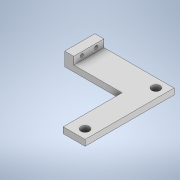
# Autodesk Inventor part: limit_switch_lower_mount
Saved by Autodesk Inventor 2022 (Build 260153000, 153)
## iProperties
Created: 2022-02-08
Part Number: limit_switch_lower_mount
Material: Generic
Document SubType Name: Modeling
Designer: kylem
Density: 1 g/cm^3
Appearance: Default
Author: kylem
Autodesk Inventor part; units mm, degrees
ref_plane "YZ Plane" through (0, 0, 0) normal (1, 0, 0) x (0, 1, 0)
ref_plane "XZ Plane" through (0, 0, 0) normal (0, 1, 0) x (-1, 0, 0)
ref_plane "XY Plane" through (0, 0, 0) normal (0, 0, 1) x (1, 0, 0)
sketch "Sketch1" plane through (0, 0, 0) normal (0, 1, 0) x (-1, 0, 0)
  line L0 (0, 0) -> (40.5, 0)
  line L1 (40.5, 0) -> (40.5, -47)
  line L2 (40.5, -47) -> (0, -47)
  line L3 (0, -47) -> (0, 0)
  circle A0 centre (0, 0) radius 2.8
  circle A1 centre (0, -47) radius 2.8
  line L4 (0, 0) -> (-6, 0)
  line L5 (-6, 0) -> (-6, 6)
  line L6 (0, -47) -> (-6, -47)
  line L7 (-6, -47) -> (-6, -53)
  line L8 (-6, -53) -> (40.5, -53)
  line L9 (40.5, -53) -> (-6, -53)
  line L10 (-6, -53) -> (-6, 6)
  line L11 (-6, 6) -> (40.5, 6)
  line L12 (40.5, 6) -> (40.5, -53)
  line L13 (40.5, 6) -> (46.5, 6)
  line L14 (46.5, 6) -> (46.5, -53)
  line L15 (46.5, -53) -> (40.5, -53)
  line L16 (40.5, -53) -> (40.5, 6)
  dimension "d0" = 40.5
  dimension "d1" = 47
  dimension "d2" = 5.6
  dimension "d3" = 5.6
  dimension "d4" = 6
  dimension "d5" = 6
  dimension "d6" = 6
  dimension "d7" = 6
  dimension "d8" = 6
  constraints: 34 end point, 7 perpendicular, 6 parallel, 4 horizontal, 2 centre point, 2 coincident, 1 point on line
  measures "d0" distance of L1.end L2.end
  measures "d1" distance of L0.end L1.end
  measures "d2" diameter of A0
  measures "d3" diameter of A1
  measures "d4" distance of L4.start L4.end
  measures "d5" distance of L4.end L5.end
  measures "d6" distance of L6.start L6.end
  measures "d7" distance of L6.end L7.end
  measures "d8" distance of L14.end L15.end
extrude "Extrusion1" add sketch "Sketch1" along normal blind 4 contours A0 L4 L5 L11 L12 L0 | L0 L1 L2 A1 L3 A0 | L3 A1 L6 L10 L4 A0 | L12 L13 L14 L15 L1 | L12 L8 L7 L6 A1 L2
sketch "Sketch3" plane through (-46.5, 0, -53) normal (-1, 0, 0) x (0, 0, 1)
  line L0 (0, 0) -> (0, 4) projected
  line L1 (0, 4) -> (20, 4)
  line L2 (20, 4) -> (20, 9)
  line L3 (20, 9) -> (0, 9)
  line L4 (0, 9) -> (0, 4)
  point P0 (53, 0)
  dimension "d11" = 20
  dimension "d12" = 5
  constraints: 8 end point, 2 parallel, 1 horizontal, 1 perpendicular
  measures "d11" distance of L3.end L2.end
  measures "d12" distance of L2.end L1.end
extrude "Extrusion2" add sketch "Sketch3" against normal blind 6
sketch "Sketch4" plane through (0, 4, 0) normal (0, 1, 0) x (1, 0, 0)
  line L0 (-46.5, -6) -> (6, -6) projected
  line L1 (-46.5, -6) -> (-8.5, -6)
  line L2 (-8.5, -6) -> (-8.5, 36)
  line L3 (-8.5, 36) -> (-46.5, 36)
  line L4 (-46.5, 36) -> (-46.5, -6)
  point P0 (0, 0)
  dimension "d15" = 38
  dimension "d16" = 42
  constraints: 8 end point, 2 parallel, 1 horizontal, 1 perpendicular
  measures "d15" distance of L3.end L2.end
  measures "d16" distance of L2.end L1.end
extrude "Extrusion3" cut sketch "Sketch4" against normal blind 6
sketch "Sketch5" plane through (-46.5, 9, -53) normal (-1, 0, 0) x (0, 0, 1)
  line L0 (20, 0) -> (0, 0) projected
  line L1 (10, 0) -> (5.25, 0)
  line L2 (5.25, 0) -> (5.25, 2.25)
  line L3 (5.25, 0) -> (5.25, -2.25)
  line L4 (5.25, -2.25) -> (14.75, -2.25)
  circle A0 centre (5.25, -2.25) radius 1.1
  circle A1 centre (14.75, -2.25) radius 1.1
  point P0 (53, -9)
  dimension "d19" = 4.75
  dimension "d20" = 2.25
  dimension "d21" = 90
  dimension "d22" = 2.25
  dimension "d23" = 9.5
  dimension "d24" = 2.2
  dimension "d25" = 2.2
  constraints: 8 end point, 2 centre point, 2 coincident, 2 perpendicular, 1 midpoint, 1 point on line, 1 vertical
  measures "d19" distance of L1.start L1.end
  measures "d20" distance of L1.end L2.end
  measures "d21" angle of L1 L2
  measures "d22" distance of L1.end L3.end
  measures "d23" distance of L3.end L4.end
  measures "d24" diameter of A0
  measures "d25" diameter of A1
extrude "Extrusion4" cut sketch "Sketch5" against normal blind 6
sketch "Sketch6" plane through (0, 4, 0) normal (0, -1, 0) x (1, 0, 0)
  line L0 (-46.5, -36) -> (-46.5, -33) projected
  line L1 (-8.5, -36) -> (-8.5, 6) projected
  line L2 (-46.5, -33) -> (-8.5, -33)
  line L3 (-8.5, -33) -> (-8.5, -36)
  line L4 (-8.5, -36) -> (-46.5, -36)
  line L5 (-46.5, -36) -> (-46.5, -33)
  point P0 (0, 0)
  constraints: 8 end point, 2 parallel, 1 horizontal, 1 perpendicular
extrude "Extrusion5" add sketch "Sketch6" along normal blind 4
body "Solid1"
